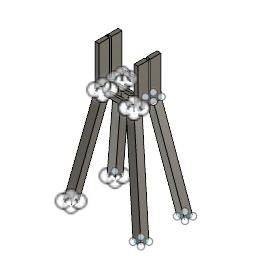
sht40_holder_v1 (Autodesk Fusion 360 design; units mm, degrees)
part number: 2026-08-17-11-59-10-058
Autodesk Fusion 360 part; units mm, degrees
ref_plane "WorkPlane1" through (0, 0, 100) normal (0, 0, 1) x (1, 0, 0)
ref_plane "WorkPlane2" through (0, 0, 100) normal (0, 0, 1) x (1, 0, 0)
ref_plane "WorkPlane3" through (0, 0, 100) normal (0, 0, 1) x (1, 0, 0)
ref_plane "WorkPlane4" through (0, 0, 100) normal (0, 0, 1) x (1, 0, 0)
ref_plane "WorkPlane5" through (0, 0, 100) normal (0, 0, 1) x (1, 0, 0)
ref_plane "WorkPlane6" through (0, 0, 100) normal (0, 0, 1) x (1, 0, 0)
ref_plane "WorkPlane7" through (0, 0, 100) normal (0, 0, 1) x (1, 0, 0)
ref_plane "WorkPlane8" through (0, 0, 100) normal (0, 0, 1) x (1, 0, 0)
ref_plane "WorkPlane9" through (0, 0, 100) normal (0, 0, 1) x (1, 0, 0)
ref_plane "WorkPlane10" through (0, 0, 100) normal (0, 0, 1) x (1, 0, 0)
ref_plane "WorkPlane11" through (0, 0, 100) normal (0, 0, 1) x (1, 0, 0)
ref_plane "WorkPlane12" through (0, 0, 100) normal (0, 0, 1) x (1, 0, 0)
ref_plane "WorkPlane13" through (0, 0, 100) normal (0, 0, 1) x (1, 0, 0)
ref_plane "WorkPlane14" through (0, 0, 100) normal (0, 0, 1) x (1, 0, 0)
ref_plane "WorkPlane15" through (0, 0, 100) normal (0, 0, 1) x (1, 0, 0)
ref_plane "WorkPlane16" through (0, 0, 100) normal (0, 0, 1) x (1, 0, 0)
ref_plane "WorkPlane18" through (0, 0, 100) normal (0, 0, 1) x (1, 0, 0)
ref_plane "WorkPlane20" through (0, 0, 100) normal (0, 0, 1) x (1, 0, 0)
ref_plane "WorkPlane21" through (0, 0, 105) normal (0, 0, 1) x (1, 0, 0)
ref_plane "WorkPlane22" through (0, 0, 100) normal (0, 0, 1) x (1, 0, 0)
ref_plane "WorkPlane23" through (0, 0, 105) normal (0, 0, 1) x (1, 0, 0)
ref_plane "WorkPlane25" through (0, 0, 105) normal (0, 0, 1) x (1, 0, 0)
ref_plane "WorkPlane26" through (0, 0, 100) normal (0, 0, 1) x (1, 0, 0)
ref_plane "WorkPlane27" through (0, 0, 100) normal (0, 0, 1) x (1, 0, 0)
ref_plane "WorkPlane28" through (0, 0, 105) normal (0, 0, 1) x (1, 0, 0)
ref_plane "WorkPlane29" through (0, 0, 100) normal (0, 0, 1) x (1, 0, 0)
ref_plane "WorkPlane31" through (0, 0, 105) normal (0, 0, 1) x (1, 0, 0)
ref_plane "WorkPlane32" through (0, 0, 100) normal (0, 0, 1) x (1, 0, 0)
ref_plane "WorkPlane33" through (0, 0, 105) normal (0, 0, 1) x (1, 0, 0)
ref_plane "WorkPlane34" through (0, 0, 0) normal (0, 0, 1) x (1, 0, 0)
ref_plane "WorkPlane35" through (0, 0, 0) normal (0, 0, 1) x (1, 0, 0)
ref_plane "WorkPlane36" through (0, 0, 0) normal (0, 0, 1) x (1, 0, 0)
ref_plane "WorkPlane37" through (0, 0, 0) normal (0, 0, 1) x (1, 0, 0)
ref_plane "WorkPlane38" through (0, 0, 100) normal (0, 0, 1) x (1, 0, 0)
ref_plane "WorkPlane39" through (0, 0, 100) normal (0, 0, 1) x (1, 0, 0)
ref_plane "WorkPlane40" through (0, 0, 105) normal (0, 0, 1) x (1, 0, 0)
ref_plane "WorkPlane41" through (0, 0, 0) normal (0, 0, 1) x (1, 0, 0)
ref_plane "WorkPlane42" through (0, 0, 0) normal (0, 0, 1) x (1, 0, 0)
ref_plane "WorkPlane43" through (0, 0, 0) normal (0, 0, 1) x (1, 0, 0)
ref_plane "WorkPlane44" through (0, 0, 0) normal (0, 0, 1) x (1, 0, 0)
ref_plane "WorkPlane45" through (0, 0, 100) normal (0, 0, 1) x (1, 0, 0)
ref_plane "WorkPlane46" through (0, 0, 100) normal (0, 0, 1) x (1, 0, 0)
ref_plane "WorkPlane47" through (0, 0, 100) normal (0, 0, 1) x (1, 0, 0)
ref_plane "WorkPlane48" through (0, 0, 100) normal (0, 0, 1) x (1, 0, 0)
ref_plane "WorkPlane49" through (0, 0, 0) normal (0, 0, 1) x (1, 0, 0)
ref_plane "WorkPlane50" through (0, 0, 100) normal (0, 0, 1) x (1, 0, 0)
ref_plane "WorkPlane51" through (0, 0, 0) normal (0, 0, 1) x (1, 0, 0)
ref_plane "WorkPlane52" through (0, 0, 100) normal (0, 0, 1) x (1, 0, 0)
ref_plane "WorkPlane53" through (0, 0, 0) normal (0, 0, 1) x (1, 0, 0)
ref_plane "WorkPlane54" through (0, 0, 100) normal (0, 0, 1) x (1, 0, 0)
ref_plane "WorkPlane55" through (0, 0, 0) normal (0, 0, 1) x (1, 0, 0)
ref_plane "WorkPlane56" through (0, 0, 100) normal (0, 0, 1) x (1, 0, 0)
ref_plane "WorkPlane57" through (0, 0, 100) normal (0, 0, 1) x (1, 0, 0)
ref_plane "WorkPlane58" through (0, 0, 0) normal (0, 0, 1) x (1, 0, 0)
ref_plane "WorkPlane59" through (0, 0, 100) normal (0, 0, 1) x (1, 0, 0)
sketch "Sketch240" plane through (0, 0, 0) normal (0, 0, 1) x (1, 0, 0)
  line L0 (31, 18) -> (39, 18)
  line L1 (39, 18) -> (39, 26)
  line L2 (39, 26) -> (31, 26)
  line L3 (31, 26) -> (31, 18)
sketch "Sketch241" plane through (0, 0, 100) normal (0, 0, 1) x (1, 0, 0)
  line L0 (11.7, 5.7) -> (19.7, 5.7)
  line L1 (19.7, 5.7) -> (19.7, 13.7)
  line L2 (19.7, 13.7) -> (11.7, 13.7)
  line L3 (11.7, 13.7) -> (11.7, 5.7)
loft "Loft97" add profiles "Sketch240", "Sketch241" section 1 section 2 makes body 1
ref_plane "WorkPlane60" through (0, 0, 0) normal (0, 0, 1) x (1, 0, 0)
ref_plane "WorkPlane61" through (0, 0, 100) normal (0, 0, 1) x (1, 0, 0)
sketch "Sketch242" plane through (0, 0, 0) normal (0, 0, 1) x (1, 0, 0)
  line L0 (-39, 18) -> (-31, 18)
  line L1 (-31, 18) -> (-31, 26)
  line L2 (-31, 26) -> (-39, 26)
  line L3 (-39, 26) -> (-39, 18)
sketch "Sketch243" plane through (0, 0, 100) normal (0, 0, 1) x (1, 0, 0)
  line L0 (-19.7, 5.7) -> (-11.7, 5.7)
  line L1 (-11.7, 5.7) -> (-11.7, 13.7)
  line L2 (-11.7, 13.7) -> (-19.7, 13.7)
  line L3 (-19.7, 13.7) -> (-19.7, 5.7)
loft "Loft98" add profiles "Sketch242", "Sketch243" section 1 section 2 separate body makes body 2
ref_plane "WorkPlane62" through (0, 0, 0) normal (0, 0, 1) x (1, 0, 0)
ref_plane "WorkPlane63" through (0, 0, 100) normal (0, 0, 1) x (1, 0, 0)
sketch "Sketch244" plane through (0, 0, 0) normal (0, 0, 1) x (1, 0, 0)
  line L0 (-39, -26) -> (-31, -26)
  line L1 (-31, -26) -> (-31, -18)
  line L2 (-31, -18) -> (-39, -18)
  line L3 (-39, -18) -> (-39, -26)
sketch "Sketch245" plane through (0, 0, 100) normal (0, 0, 1) x (1, 0, 0)
  line L0 (-19.7, -13.7) -> (-11.7, -13.7)
  line L1 (-11.7, -13.7) -> (-11.7, -5.7)
  line L2 (-11.7, -5.7) -> (-19.7, -5.7)
  line L3 (-19.7, -5.7) -> (-19.7, -13.7)
loft "Loft99" add profiles "Sketch244", "Sketch245" section 1 section 2 separate body makes body 3
ref_plane "WorkPlane64" through (0, 0, 0) normal (0, 0, 1) x (1, 0, 0)
ref_plane "WorkPlane65" through (0, 0, 100) normal (0, 0, 1) x (1, 0, 0)
sketch "Sketch246" plane through (0, 0, 0) normal (0, 0, 1) x (1, 0, 0)
  line L0 (31, -26) -> (39, -26)
  line L1 (39, -26) -> (39, -18)
  line L2 (39, -18) -> (31, -18)
  line L3 (31, -18) -> (31, -26)
sketch "Sketch247" plane through (0, 0, 100) normal (0, 0, 1) x (1, 0, 0)
  line L0 (11.7, -13.7) -> (19.7, -13.7)
  line L1 (19.7, -13.7) -> (19.7, -5.7)
  line L2 (19.7, -5.7) -> (11.7, -5.7)
  line L3 (11.7, -5.7) -> (11.7, -13.7)
loft "Loft100" add profiles "Sketch246", "Sketch247" section 1 section 2 separate body makes body 4
ref_plane "WorkPlane66" through (0, 0, 100) normal (0, 0, 1) x (1, 0, 0)
sketch "Sketch248" plane through (0, 0, 100) normal (0, 0, 1) x (1, 0, 0)
  line L0 (-19.7, -13.7) -> (19.7, -13.7)
  line L1 (19.7, -13.7) -> (19.7, 13.7)
  line L2 (19.7, 13.7) -> (-19.7, 13.7)
  line L3 (-19.7, 13.7) -> (-19.7, -13.7)
  line L4 (-17.5, -11.5) -> (17.5, -11.5)
  line L5 (17.5, -11.5) -> (17.5, 11.5)
  line L6 (17.5, 11.5) -> (-17.5, 11.5)
  line L7 (-17.5, 11.5) -> (-17.5, -11.5)
extrude "Extrude50" add sketch "Sketch248" along normal blind 5 bodies 1 2 3 4
ref_plane "WorkPlane67" through (0, 0, 105.1) normal (0, 0, 1) x (1, 0, 0)
sketch "sk_CutInner" plane through (0, 0, 105.1) normal (0, 0, 1) x (1, 0, 0)
  line L0 (-17.4, -11.4) -> (17.4, -11.4)
  line L1 (17.4, -11.4) -> (17.4, 11.4)
  line L2 (17.4, 11.4) -> (-17.4, 11.4)
  line L3 (-17.4, 11.4) -> (-17.4, -11.4)
extrude "Extrude51" cut sketch "sk_CutInner" against normal blind 5.7 bodies 1
sketch "sk_RailRight" plane through (0, 0, 0) normal (0, 0, 1) x (1, 0, 0)
  line L0 (17.5, -11.5) -> (21.5, -11.5)
  line L1 (21.5, -11.5) -> (21.5, 11.5)
  line L2 (21.5, 11.5) -> (17.5, 11.5)
  line L3 (17.5, 11.5) -> (17.5, -11.5)
extrude "Extrude52" add sketch "sk_RailRight" along normal blind 140 separate body makes body 5
sketch "sk_GrooveRight" plane through (0, 0, 0) normal (0, 0, 1) x (1, 0, 0)
  line L0 (17.5, -1.1) -> (21, -1.1)
  line L1 (21, -1.1) -> (21, 1.1)
  line L2 (21, 1.1) -> (17.5, 1.1)
  line L3 (17.5, 1.1) -> (17.5, -1.1)
extrude "Extrude53" cut sketch "sk_GrooveRight" along normal blind 140 bodies 5
sketch "sk_TrimRailRight" plane through (0, 0, 0) normal (0, 0, 1) x (1, 0, 0)
  line L0 (17.5, -11.5) -> (21.5, -11.5)
  line L1 (21.5, -11.5) -> (21.5, 11.5)
  line L2 (21.5, 11.5) -> (17.5, 11.5)
  line L3 (17.5, 11.5) -> (17.5, -11.5)
extrude "Extrude54" cut sketch "sk_TrimRailRight" along normal blind 100 bodies 5
sketch "sk_RailLeft" plane through (0, 0, 0) normal (0, 0, 1) x (1, 0, 0)
  line L0 (-21.5, -11.5) -> (-17.5, -11.5)
  line L1 (-17.5, -11.5) -> (-17.5, 11.5)
  line L2 (-17.5, 11.5) -> (-21.5, 11.5)
  line L3 (-21.5, 11.5) -> (-21.5, -11.5)
extrude "Extrude55" add sketch "sk_RailLeft" along normal blind 140 separate body makes body 6
sketch "sk_GrooveLeft" plane through (0, 0, 0) normal (0, 0, 1) x (1, 0, 0)
  line L0 (-21, -1.1) -> (-17.5, -1.1)
  line L1 (-17.5, -1.1) -> (-17.5, 1.1)
  line L2 (-17.5, 1.1) -> (-21, 1.1)
  line L3 (-21, 1.1) -> (-21, -1.1)
extrude "Extrude56" cut sketch "sk_GrooveLeft" along normal blind 140 bodies 6
sketch "sk_TrimRailLeft" plane through (0, 0, 0) normal (0, 0, 1) x (1, 0, 0)
  line L0 (-21.5, -11.5) -> (-17.5, -11.5)
  line L1 (-17.5, -11.5) -> (-17.5, 11.5)
  line L2 (-17.5, 11.5) -> (-21.5, 11.5)
  line L3 (-21.5, 11.5) -> (-21.5, -11.5)
extrude "Extrude57" cut sketch "sk_TrimRailLeft" along normal blind 100 bodies 6
sketch "sk_BottomStop" plane through (0, 0, 0) normal (0, 0, 1) x (1, 0, 0)
  line L0 (-17.5, -1.2) -> (17.5, -1.2)
  line L1 (17.5, -1.2) -> (17.5, 1.2)
  line L2 (17.5, 1.2) -> (-17.5, 1.2)
  line L3 (-17.5, 1.2) -> (-17.5, -1.2)
extrude "Extrude58" add sketch "sk_BottomStop" along normal blind 103 separate body makes body 7
sketch "sk_TrimStop" plane through (0, 0, 0) normal (0, 0, 1) x (1, 0, 0)
  line L0 (-17.5, -1.2) -> (17.5, -1.2)
  line L1 (17.5, -1.2) -> (17.5, 1.2)
  line L2 (17.5, 1.2) -> (-17.5, 1.2)
  line L3 (-17.5, 1.2) -> (-17.5, -1.2)
extrude "Extrude59" cut sketch "sk_TrimStop" along normal blind 100 bodies 7
combine "Combine1" operation add target body 1 tool bodies 5 6 7
named bodies: "RailRight", "RailLeft", "BottomStop"
